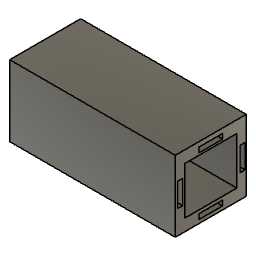
DiffusorTestor v1 (Autodesk Fusion 360 design; units mm, degrees)
Autodesk Fusion 360 part; units mm, degrees
sketch "Sketch1" plane through (0, 0, 0) normal (1, 0, 0) x (0, 1, 0)
  line L0 (0, 0) -> (30, 0)
  line L1 (30, 0) -> (30, 30)
  line L2 (30, 30) -> (0, 30)
  line L3 (0, 30) -> (0, 0)
  line L4 (1, 20) -> (3.1, 20)
  line L5 (3.1, 20) -> (3.1, 10)
  line L6 (3.1, 10) -> (1, 10)
  line L7 (1, 10) -> (1, 20)
  line L8 (10, 28) -> (20, 28)
  line L9 (20, 28) -> (20, 25.9)
  line L10 (20, 25.9) -> (10, 25.9)
  line L11 (10, 25.9) -> (10, 28)
  line L12 (29.5, 19.9621) -> (27.4, 19.9621)
  line L13 (27.4, 19.9621) -> (27.4, 9.9621)
  line L14 (27.4, 9.9621) -> (29.5, 9.9621)
  line L15 (29.5, 9.9621) -> (29.5, 19.9621)
  line L16 (10, 1.5) -> (20, 1.5)
  line L17 (20, 1.5) -> (20, 3.6)
  line L18 (20, 3.6) -> (10, 3.6)
  line L19 (10, 3.6) -> (10, 1.5)
  line L20 (4, 25) -> (26, 25)
  line L21 (26, 25) -> (26, 5)
  line L22 (26, 5) -> (4, 5)
  line L23 (4, 5) -> (4, 25)
  dimension "d1" = 30
  dimension "d2" = 30
  dimension "d3" = 2.1
  dimension "d4" = 10
  dimension "d5" = 10
  dimension "d6" = 2.1
  dimension "d7" = 2.1
  dimension "d8" = 10
  dimension "d9" = 0.5
  dimension "d10" = 10
  dimension "d11" = 2.1
  dimension "d12" = 1.5
  constraint horizontal L0
  constraint vertical L1
  constraint horizontal L2
  constraint vertical L3
  constraint coincident L0.start L3.end
  constraint horizontal L4
  constraint vertical L5
  constraint horizontal L6
  constraint vertical L7
  constraint horizontal L8
  constraint vertical L9
  constraint horizontal L10
  constraint vertical L11
  constraint horizontal L12
  constraint vertical L13
  constraint horizontal L14
  constraint vertical L15
  constraint horizontal L16
  constraint vertical L17
  constraint horizontal L18
  constraint vertical L19
  constraint horizontal L20
  constraint vertical L21
  constraint horizontal L22
  constraint vertical L23
  measures "d1" distance of L0.start L0.end
  measures "d2" distance of L0.start L2.end
  measures "d3" distance of L4.start L4.end
  measures "d4" distance of L4.start L6.end
  measures "d5" distance of L8.start L8.end
  measures "d6" distance of L8.start L10.end
  measures "d7" distance of L12.start L12.end
  measures "d8" distance of L12.start L14.end
  measures "d9" distance of L1 L15
  measures "d10" distance of L16.start L16.end
  measures "d11" distance of L16.start L18.end
  measures "d12" distance of L0 L16
extrude "Extrude1" add sketch "Sketch1" along normal blind 70
